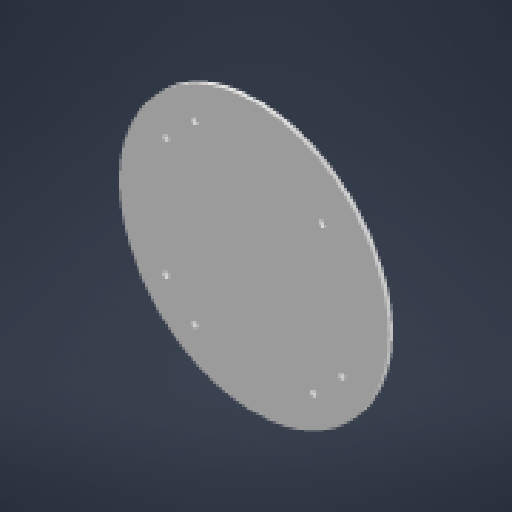
# Autodesk Inventor part: Platform
Saved by Autodesk Inventor 2026.1 (Build 301233020, 233B)
## iProperties
Created: 2026-03-09
Part Number: Platform
Material: Generic
Document SubType Name: Modeling
Designer: Mikke
Density: 1 g/cm^3
Appearance: Default
Author: Mikke
Autodesk Inventor part; units mm, degrees
ref_plane "YZ Plane" through (0, 0, 0) normal (1, 0, 0) x (0, 1, 0)
ref_plane "XZ Plane" through (0, 0, 0) normal (0, 1, 0) x (-1, 0, 0)
ref_plane "XY Plane" through (0, 0, 0) normal (0, 0, 1) x (1, 0, 0)
sketch "Sketch2" plane through (0, 0, 0) normal (0, 0, 1) x (1, 0, 0)
  arc A0 (-15.7199, 60.6781) -> (-34.0297, 78.9878) centre (-90.4651, 4.2426) ccw projected
  line L0 (-14.6737, 61.0337) -> (-15.7199, 60.6781) projected
  arc A1 (-8.1943, -42.6729) -> (-14.6737, 61.0337) centre (-90.4651, 4.2426) ccw projected
  line L1 (-8.1943, -42.6729) -> (-20.7966, -30.0705) projected
  arc A2 (-20.7966, -30.0705) -> (-27.8677, -30.0705) centre (-24.3322, -33.606) ccw projected
  line L2 (-27.8677, -30.0705) -> (-56.152, -58.3548) projected
  arc A3 (-56.152, -58.3548) -> (-56.152, -65.4258) centre (-52.6165, -61.8903) ccw projected
  line L3 (-56.152, -65.4258) -> (-43.5496, -78.0282) projected
  arc A4 (-137.3806, -78.0282) -> (-43.5496, -78.0282) centre (-90.4651, 4.2426) ccw projected
  line L4 (-137.3806, -78.0282) -> (-124.7782, -65.4258) projected
  arc A5 (-124.7782, -65.4258) -> (-124.7782, -58.3548) centre (-128.3138, -61.8903) ccw projected
  line L5 (-124.7782, -58.3548) -> (-153.0625, -30.0705) projected
  arc A6 (-153.0625, -30.0705) -> (-160.1336, -30.0705) centre (-156.598, -33.606) ccw projected
  line L6 (-160.1336, -30.0705) -> (-172.736, -42.6729) projected
  arc A7 (-172.736, 51.1582) -> (-172.736, -42.6729) centre (-90.4651, 4.2426) ccw projected
  line L7 (-172.736, 51.1582) -> (-160.1336, 38.5558) projected
  arc A8 (-160.1336, 38.5558) -> (-153.0625, 38.5558) centre (-156.598, 42.0913) ccw projected
  line L8 (-153.0625, 38.5558) -> (-124.7782, 66.84) projected
  arc A9 (-124.7782, 66.84) -> (-124.7782, 73.9111) centre (-128.3138, 70.3756) ccw projected
  line L9 (-124.7782, 73.9111) -> (-137.3806, 86.5135) projected
  arc A10 (-33.674, 80.034) -> (-137.3806, 86.5135) centre (-90.4651, 4.2426) ccw projected
  line L10 (-34.0297, 78.9878) -> (-33.674, 80.034) projected
  circle A11 centre (-90.4651, 4.2426) radius 98.723 projected
  circle A12 centre (-133.9706, -60.4761) radius 2.25 projected
  circle A13 centre (-155.1838, -39.2629) radius 2.25 projected
  circle A14 centre (-155.1838, 47.7482) radius 2.25 projected
  circle A15 centre (-133.9706, 68.9614) radius 2.25 projected
  circle A16 centre (-46.9596, -60.4761) radius 2.25 projected
  circle A17 centre (-25.7464, -39.2629) radius 2.25 projected
  circle A18 centre (-52.9194, 36.1773) radius 1.5 projected
  circle A19 centre (-30.999, 58.0977) radius 1.5 projected
  circle A20 centre (-52.9194, 58.0977) radius 2.5 projected
  circle A21 centre (-74.8397, 58.0977) radius 1.5 projected
  circle A22 centre (-52.9194, 80.018) radius 1.5 projected
  circle A23 centre (-90.4651, 4.2426) radius 98.723
  point P0 (0, 0)
  constraints: 1 centre point, 1 coincident, 1 concentric
extrude "Extrusion2" add sketch "Sketch2" along normal blind 3 contours L0 A1 L1 A2 L2 A3 L3 A4 L4 A5 L5 A6 L6 A7 L7 A8 L8 A9 L9 A10 L10 A0 | A11
sketch "Sketch3" plane through (-90.4651, 4.2426, 3) normal (0, 0, 1) x (1, 0, 0)
  line L0 (-50, 0) -> (-50, -50)
  line L1 (-50, -50) -> (0, -50)
  circle A0 centre (-50, -50) radius 1.75
  point P0 (90.4651, -4.2426)
  dimension "d6" = 50
  dimension "d7" = 50
  dimension "d8" = 3.5
  constraints: 4 end point, 1 centre point, 1 coincident
  measures "d6" distance of L1.end L0.end
  measures "d7" distance of L0.end L0.start
  measures "d8" diameter of A0
extrude "Extrusion3" cut sketch "Sketch3" against normal blind 3
pattern_linear "Rectangular Pattern1" count 11 spacing 10 along (0, 1, 0) count 6 spacing 10 along (1, 0, 0) of "Extrusion3"
pattern_linear "Rectangular Pattern2" count 6 spacing 10 along (0, 1, 0) count 11 spacing 10 along (1, 0, 0) of "Extrusion3"
sketch "Sketch4" plane through (-90.4651, 4.2426, 3) normal (0, 0, 1) x (1, 0, 0)
  circle A0 centre (-30, -50) radius 1.75 projected
  line L0 (-30, -50) -> (-30, -60)
  line L1 (-30, -50) -> (-20, -50) construction
  line L2 (-30, -60) -> (-30, -70)
  line L3 (-30, -70) -> (-30, -80)
  circle A1 centre (-30, -80) radius 1.75
  point P0 (90.4651, -4.2426)
  dimension "d23" = 10
  dimension "d24" = 90
  dimension "d28" = 10
  dimension "d29" = 10
  dimension "d30" = 3.5
  constraints: 8 end point, 2 coincident, 2 vertical, 1 centre point, 1 horizontal, 1 perpendicular, 1 point on line
  measures "d23" distance of L0.start L0.end
  measures "d24" angle of L0 L1
  measures "d28" distance of L2.start L2.end
  measures "d29" distance of L2.end L3.end
  measures "d30" diameter of A1
extrude "Extrusion4" cut sketch "Sketch4" against normal blind 3 contours A1
pattern_linear "Rectangular Pattern3" count 3 spacing 10 along (0, 1, 0) count 7 spacing 10 along (1, 0, 0) of "Extrusion4"
sketch "Sketch5" plane through (-90.4651, 4.2426, 3) normal (0, 0, 1) x (1, 0, 0)
  circle A0 centre (-50, -30) radius 1.75 projected
  line L0 (-50, -30) -> (-80, -30)
  circle A1 centre (-80, -30) radius 1.75
  point P0 (90.4651, -4.2426)
  dimension "d37" = 30
  dimension "d38" = 3.5
  constraints: 2 end point, 1 centre point, 1 coincident, 1 horizontal
  measures "d37" distance of L0.start L0.end
  measures "d38" diameter of A1
extrude "Extrusion5" cut sketch "Sketch5" against normal blind 3 contours A1
pattern_linear "Rectangular Pattern4" count 7 spacing 10 along (0, 1, 0) count 3 spacing 10 along (1, 0, 0) of "Extrusion5"
body "Solid2"
